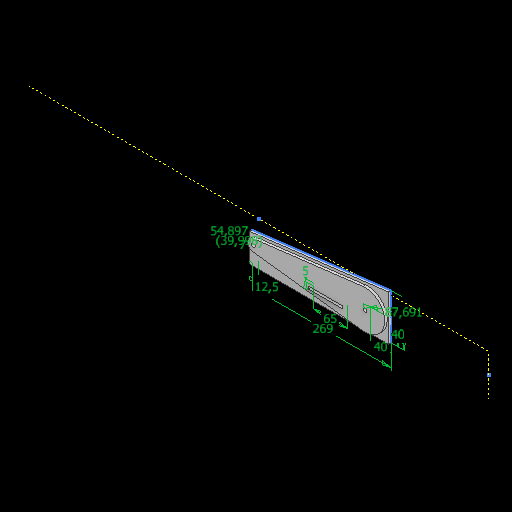
# Autodesk Inventor part: divisores_banda
Saved by Autodesk Inventor 2027 (Build 310192000, 192)
## iProperties
Created: 2026-05-13
Part Number: divisores_banda
Material: Genérico
Document SubType Name: Modeling
Designer: giova
Density: 1 g/cm^3
Appearance: Valor por defecto
Author: giova
Autodesk Inventor part; units mm, degrees
ref_plane "YZ Plane" through (0, 0, 0) normal (1, 0, 0) x (0, 1, 0)
ref_plane "XZ Plane" through (0, 0, 0) normal (0, 1, 0) x (-1, 0, 0)
ref_plane "XY Plane" through (0, 0, 0) normal (0, 0, 1) x (1, 0, 0)
sketch "Boceto1" plane through (0, 0, 0) normal (0, 0, 1) x (1, 0, 0)
  circle A0 centre (229, 39.9983) radius 35 construction
  line L0 (269, 87.6892) -> (269, -0.002)
  line L1 (269, -0.002) -> (0, 0)
  line L2 (0, 0) -> (0, 54.8968)
  line L3 (457.9938, -0.0034) -> (457.9938, 80) construction
  line L4 (457.9938, 80) -> (-432.9938, 80) construction
  line L5 (189, -0.0014) -> (189, 79.998) construction
  line L6 (189, 79.998) -> (269, 79.998) construction
  circle A1 centre (229, 39.9983) radius 11.3 construction
  line L7 (119, 54.9966) -> (199, 54.9966) construction
  line L8 (199, 54.9966) -> (199, 25) construction
  line L9 (199, 25) -> (119, 25) construction
  line L10 (119, 25) -> (119, 54.9966) construction
  arc A2 (224.4624, 2.7754) -> (224.4624, 77.2212) centre (229, 39.9983) ccw
  arc A3 (11.1326, 51.2153) -> (11.1326, 28.7814) centre (12.5, 39.9983) ccw
  line L11 (224.4624, 77.2212) -> (11.1326, 51.2153)
  line L12 (224.4624, 2.7754) -> (11.1326, 28.7814)
  line L13 (0, 54.8968) -> (269, 87.6892)
  line L14 (119, 20) -> (184, 20)
  line L15 (119, 25) -> (119, 20)
  line L16 (184, 20) -> (184, 25)
  circle A4 centre (12.5, 39.9983) radius 3.5
  circle A5 centre (229, 39.9983) radius 3.5
  circle A6 centre (229, 39.9983) radius 30 construction
  line L17 (184, 25) -> (119, 25)
  point P0 (457.9938, 39.9983)
  point P1 (12.5, 80)
  point P2 (189, 39.9983)
  point P3 (229, 79.998)
  point P4 (199, 39.9983)
  dimension "d2" = 269
  dimension "d17" = 5
  dimension "d18" = 65
  dimension "d19" = 7
  dimension "d25" = 87.6911
  dimension "d26" = 40
  dimension "d27" = 40
  dimension "d28" = 12.5
  dimension "d29" = 39.9984
  dimension "d30" = 7
  dimension "d31" = 54.8968
  constraints: 36 end point, 7 centre point, 6 coincident, 5 horizontal alignment, 5 midpoint, 5 parallel, 5 tangent, 4 perpendicular, 4 point on circle, 4 point on line, 3 vertical, 3 vertical alignment, 2 horizontal, 1 collinear
  measures "d2" distance of L0.end L1.end
  measures "d17" distance between parallel lines of L14 L9
  measures "d18" distance of L14.start L14.end
  measures "d19" diameter of A4
  measures "d25" distance of L0.start L0.end
  measures "d26" distance from line of L1 A0.centre
  measures "d27" distance from line of A0.centre L0
  measures "d28" distance from line of L2 A4.centre
  measures "d29" distance from line of L1 A3.centre
  measures "d30" diameter of A5
  measures "d31" distance of L1.end L2.end
extrude "Extrusión1" add sketch "Boceto1" along normal blind 5 contours L0 L1 L2 L13 | L12 A3 L11 A2
extrude "Extrusión2" add sketch "Boceto1" along normal blind 10 contours L12 A3 L11 A2
